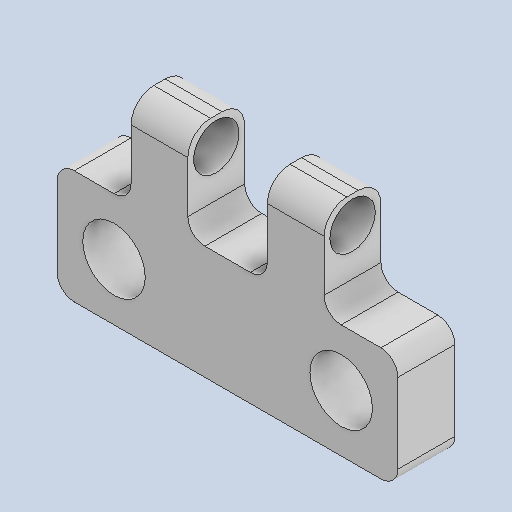
# Autodesk Inventor part: axe_camera
Saved by Autodesk Inventor 2024 (Build 280153000, 153)
## iProperties
Created: 2023-03-21
Part Number: axe_camera
Material: Generic
Document SubType Name: Modeling
Designer: Thomas
Density: 1 g/cm^3
Appearance: Default
Author: Thomas
Autodesk Inventor part; units mm, degrees
ref_plane "YZ Plane" through (0, 0, 0) normal (1, 0, 0) x (0, 1, 0)
ref_plane "XZ Plane" through (0, 0, 0) normal (0, 1, 0) x (-1, 0, 0)
ref_plane "XY Plane" through (0, 0, 0) normal (0, 0, 1) x (1, 0, 0)
sketch "Sketch1" plane through (0, 0, 0) normal (0, 0, 1) x (1, 0, 0)
  line L0 (-15, -5) -> (15, -5)
  line L1 (15, -5) -> (15, 5)
  line L2 (15, 5) -> (-15, 5)
  line L3 (-15, 5) -> (-15, -5)
  line L4 (-15, -5) -> (15, 5) construction
  line L5 (15, -5) -> (-15, 5) construction
  line L6 (-8.5, 5) -> (-8.5, 13)
  line L7 (-8.5, 13) -> (-3.5, 13)
  line L8 (-3.5, 13) -> (-3.5, 5)
  line L9 (0, 0) -> (0, 10.7683) construction
  line L10 (8.5, 5) -> (8.5, 13)
  line L11 (8.5, 13) -> (3.5, 13)
  line L12 (3.5, 13) -> (3.5, 5)
  point P0 (8.5, 5)
  point P1 (3.5, 5)
  dimension "d0" = 10
  dimension "d1" = 30
  dimension "d2" = 5
  dimension "d3" = 8
  dimension "d4" = 7
  constraints: 26 end point, 4 symmetric about line, 3 perpendicular, 2 midpoint, 2 parallel, 2 point on line, 2 vertical, 1 horizontal
  measures "d0" distance of L0.end L1.end
  measures "d1" distance of L0.start L0.end
  measures "d2" distance of L6.end L7.end
  measures "d3" distance of L6.start L6.end
  measures "d4" diameter of L8 L9
extrude "Extrusion1" add sketch "Sketch1" along normal blind 5
sketch "Sketch2" plane through (8.5, 5, 0) normal (1, 0, 0) x (0, 0, -1)
  line L0 (0, 0) -> (0, 8) projected
  line L1 (-5, 0) -> (-5, 8) projected
  line L2 (0, 8) -> (-5, 8) projected
  line L3 (0, 0) -> (-5, 0) projected
  point P0 (0, -5)
  point P1 (-2.5, 5.6)
  dimension "d14" = 2.5
  dimension "d15" = 5
  dimension "d16" = 2.4
  dimension "d17" = 8
  measures "d14" distance from line of L0 point (-2.5, 5.6)
  measures "d15" distance between parallel lines of L1 L0
  measures "d16" distance from line of point (-2.5, 5.6) L2
  measures "d17" distance between parallel lines of L3 L2
hole "Hole1" at (8.5, 10.6, 2.5) direction (-1, 0, 0) diameter 4 end through all
fillet "Fillet1" radius 2 4 edges at (6, 13, 0) (6, 13, 5) (-6, 13, 0) (-6, 13, 5)
fillet "Fillet2" radius 1.5 8 edges at (-3.5, 5, 2.5) (3.5, 5, 2.5) (-8.5, 5, 2.5) (8.5, 5, 2.5) (15, 5, 2.5) (15, -5, 2.5) (-15, -5, 2.5) (-15, 5, 2.5)
sketch "Sketch3" plane through (0, 0, 5) normal (0, 0, 1) x (1, 0, 0)
  point P0 (0, 0)
  point P1 (-10, 0)
  point P2 (10, 0)
  dimension "d27" = 10
  dimension "d30" = 360
  constraints: 1 horizontal alignment, 3 other
  measures "d27" distance of point (-10, 0) point (0, 0)
hole "Hole2" at (-10, 0, 5) at (10, 0, 5) direction (0, 0, -1) diameter 5.5 end through all clearance for "Countersunk Flat Head Screw ISO 2009/7046" size "M5" standard "ISO"
equation "\"d14\" = 0.5 * d15"
body "Solid1"
